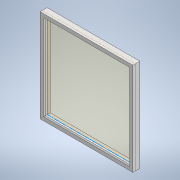
# Autodesk Inventor part: rama
Saved by Autodesk Inventor 2021 (Build 250183000, 183)
## iProperties
Created: 2021-06-22
Part Number: rama
Material: Tworzywo sztuczne PC/ABS
Document SubType Name: Modeling
Designer: Wojciech Wołczek
Density: 0.357273 g/cm^3
Appearance: Gładki — biały
Author: Wojciech Wołczek
Autodesk Inventor part; units mm, degrees
ref_plane "YZ Plane" through (0, 0, 0) normal (1, 0, 0) x (0, 1, 0)
ref_plane "XZ Plane" through (0, 0, 0) normal (0, 1, 0) x (-1, 0, 0)
ref_plane "XY Plane" through (0, 0, 0) normal (0, 0, 1) x (1, 0, 0)
sketch "Szkic1" plane through (0, 0, 0) normal (0, 0, 1) x (1, 0, 0)
  line L0 (500, -500) -> (-500, -500)
  line L1 (-500, -500) -> (-500, 500)
  line L2 (-500, 500) -> (500, 500)
  line L3 (500, 500) -> (500, -500)
  line L4 (500, -500) -> (-500, 500) construction
  line L5 (-500, -500) -> (500, 500) construction
  line L6 (465, -465) -> (-465, -465)
  line L7 (-465, -465) -> (-465, 465)
  line L8 (-465, 465) -> (465, 465)
  line L9 (465, 465) -> (465, -465)
  line L10 (465, -465) -> (-465, 465) construction
  line L11 (-465, -465) -> (465, 465) construction
  point P0 (0, 0)
  dimension "d0" = 1000
  dimension "d1" = 1000
  dimension "d2" = 930
  dimension "d3" = 930
  constraints: 24 end point, 4 midpoint, 4 parallel, 2 horizontal, 2 perpendicular
  measures "d0" distance of L1.end L2.end
  measures "d1" distance of L0.end L1.end
  measures "d2" distance of L7.end L8.end
  measures "d3" distance of L6.end L7.end
extrude "Wyciągnięcie proste1" add sketch "Szkic1" along normal mid plane 75
sketch "Szkic2" plane through (0, 0, 37.5) normal (0, 0, 1) x (1, 0, 0)
  line L0 (465, -465) -> (465, 465) projected
  line L1 (-465, 465) -> (465, 465)
  line L2 (465, 465) -> (465, -465)
  line L3 (465, -465) -> (-465, -465)
  line L4 (-465, -465) -> (-465, 465)
  line L5 (-465, 465) -> (465, -465) construction
  line L6 (465, 465) -> (-465, -465) construction
  line L7 (-452.5, 452.5) -> (452.5, 452.5)
  line L8 (452.5, 452.5) -> (452.5, -452.5)
  line L9 (452.5, -452.5) -> (-452.5, -452.5)
  line L10 (-452.5, -452.5) -> (-452.5, 452.5)
  line L11 (-452.5, 452.5) -> (452.5, -452.5) construction
  line L12 (452.5, 452.5) -> (-452.5, -452.5) construction
  point P0 (0, 0)
  dimension "d6" = 905
  dimension "d7" = 905
  constraints: 24 end point, 4 midpoint, 4 parallel, 2 horizontal, 2 perpendicular
  measures "d6" distance of L8.end L9.end
  measures "d7" distance of L7.end L8.end
extrude "Wyciągnięcie proste2" add sketch "Szkic2" against normal blind 10
chamfer "Faza1" distance 10 angle 45 4 edges at (452.5, 0, 37.5) (0, 452.5, 37.5) (-452.5, 0, 37.5) (0, -452.5, 37.5)
ref_plane "Płaszczyzna konstrukcyjna1" through (-452.5, 452.5, 27.5) normal (0, 0, 1) x (0, -1, 0)
sketch "Szkic3" plane through (0, 0, 27.5) normal (0, 0, -1) x (-1, 0, 0)
  line L0 (452.5, 452.5) -> (452.5, -452.5) projected
  line L1 (-452.5, -452.5) -> (452.5, -452.5)
  line L2 (452.5, -452.5) -> (452.5, 452.5)
  line L3 (452.5, 452.5) -> (-452.5, 452.5)
  line L4 (-452.5, 452.5) -> (-452.5, -452.5)
  line L5 (-452.5, -452.5) -> (452.5, 452.5) construction
  line L6 (452.5, -452.5) -> (-452.5, 452.5) construction
  line L7 (-457.5, -457.5) -> (457.5, -457.5)
  line L8 (457.5, -457.5) -> (457.5, 457.5)
  line L9 (457.5, 457.5) -> (-457.5, 457.5)
  line L10 (-457.5, 457.5) -> (-457.5, -457.5)
  line L11 (-457.5, -457.5) -> (457.5, 457.5) construction
  line L12 (457.5, -457.5) -> (-457.5, 457.5) construction
  point P0 (0, 0)
  dimension "d13" = 915
  constraints: 24 end point, 4 midpoint, 4 parallel, 2 horizontal, 2 perpendicular, 1 point on line
  measures "d13" distance of L9.end L8.end
extrude "Wyciągnięcie proste3" add sketch "Szkic3" along normal blind 5
